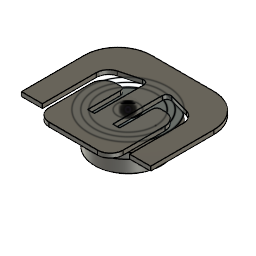
eversweet_pro_3_uvc_base (Autodesk Fusion 360 archive; units mm, degrees)
design "Kitchen Scale Load Cell"
Autodesk Fusion 360 part; units mm, degrees
sketch "Cell" plane through (0, 0, 0) normal (0, 0, 1) x (1, 0, 0)
  line L0 (0, 13) -> (7.4, 13)
  line L1 (15.4, 5) -> (15.4, -10)
  arc A0 (15.4, 5) -> (7.4, 13) centre (7.4, 5) ccw
  line L2 (15.4, -10) -> (10.4, -10)
  line L3 (10.4, -10) -> (10.4, 2.8041)
  line L4 (8.1765, 5.7018) -> (3.4588, 6.9659)
  line L5 (2.2, 6) -> (2.2, -5.8)
  line L6 (2.2, -5.8) -> (3.8, -5.8)
  line L7 (3.8, -5.8) -> (3.8, 2)
  line L8 (4.8, 3) -> (5.8, 3)
  line L9 (8.8, 0) -> (8.8, -10)
  line L10 (5.8, -13) -> (0, -13)
  line L11 (0, -25.6474) -> (0, 25.6474) construction
  arc A1 (10.4, 2.8041) -> (8.1765, 5.7018) centre (7.4, 2.8041) ccw
  arc A2 (5.8, -13) -> (8.8, -10) centre (5.8, -10) ccw
  arc A3 (8.8, 0) -> (5.8, 3) centre (5.8, 0) ccw
  arc A4 (4.8, 3) -> (3.8, 2) centre (4.8, 2) ccw
  arc A5 (3.4588, 6.9659) -> (2.2, 6) centre (3.2, 6) ccw
  line L12 (-5.8, -13) -> (0, -13)
  arc A6 (-8.8, -10) -> (-5.8, -13) centre (-5.8, -10) ccw
  line L13 (-8.8, 0) -> (-8.8, -10)
  arc A7 (-5.8, 3) -> (-8.8, 0) centre (-5.8, 0) ccw
  line L14 (-4.8, 3) -> (-5.8, 3)
  arc A8 (-3.8, 2) -> (-4.8, 3) centre (-4.8, 2) ccw
  line L15 (-3.8, -5.8) -> (-3.8, 2)
  line L16 (-2.2, -5.8) -> (-3.8, -5.8)
  line L17 (-2.2, 6) -> (-2.2, -5.8)
  arc A9 (-2.2, 6) -> (-3.4588, 6.9659) centre (-3.2, 6) ccw
  line L18 (-8.1765, 5.7018) -> (-3.4588, 6.9659)
  arc A10 (-8.1765, 5.7018) -> (-10.4, 2.8041) centre (-7.4, 2.8041) ccw
  line L19 (-10.4, -10) -> (-10.4, 2.8041)
  line L20 (-15.4, -10) -> (-10.4, -10)
  line L21 (-15.4, 5) -> (-15.4, -10)
  arc A11 (-7.4, 13) -> (-15.4, 5) centre (-7.4, 5) ccw
  line L22 (0, 13) -> (-7.4, 13)
  dimension "d3" = 8
  dimension "d4" = 5
  dimension "d7" = 26
  dimension "d8" = 16
  dimension "d9" = 1.6
  dimension "d10" = 1.6
  dimension "d12" = 7.2
  dimension "d13" = 23
  dimension "d14" = 3
  dimension "d15" = 3
  dimension "d16" = 3
  dimension "d17" = 1
  dimension "d18" = 1
  dimension "d19" = 7
  dimension "d20" = 13
  dimension "d21" = 75
  dimension "d22" = 2.2
  dimension "d23" = 5
  constraint horizontal L0
  constraint perpendicular L0 L1
  constraint tangent L0 A0
  constraint tangent L1 A0
  constraint perpendicular L1 L2
  constraint perpendicular L2 L3
  constraint perpendicular L2 L5
  constraint perpendicular L5 L6
  constraint perpendicular L6 L7
  constraint perpendicular L7 L8
  constraint perpendicular L8 L9
  constraint perpendicular L9 L10
  constraint vertical L11
  constraint coincident origin L11
  constraint midpoint origin L11
  constraint coincident L0.start L11
  constraint coincident L10.end L11
  constraint tangent L3 A1
  constraint tangent L4 A1
  constraint tangent L9 A2
  constraint tangent L10 A2
  constraint tangent L8 A3
  constraint tangent L9 A3
  constraint tangent L7 A4
  constraint tangent L8 A4
  constraint tangent L4 A5
  constraint tangent L5 A5
  constraint symmetric L1.end L11 L20.start
  constraint symmetric L0.start L11 L22.start
  constraint symmetric L0.end L11 A11.start
  constraint symmetric L1.start L11 L21.start
  constraint symmetric A0 L11 A11
  constraint symmetric L2.end L11 L19.start
  constraint symmetric L5.end L11 L16.start
  constraint symmetric L6.end L11 L15.start
  constraint symmetric L10.end L11 L12.end
  constraint symmetric L11 L3.end A10.end
  constraint symmetric L11 L4.start L18.start
  constraint symmetric L11 A1 A10
  constraint symmetric L11 L9.end A6.start
  constraint symmetric L11 L10.start L12.start
  constraint symmetric L11 A2 A6
  constraint symmetric L11 L8.end A7.start
  constraint symmetric L11 L9.start L13.start
  constraint symmetric L11 A3 A7
  constraint symmetric L11 L7.end A8.start
  constraint symmetric L11 L8.start L14.start
  constraint symmetric L11 A4 A8
  constraint symmetric L11 L4.end A9.end
  constraint symmetric L11 L5.start L17.start
  constraint symmetric L11 A5 A9
  measures "d3" radius of A0
  measures "d4" distance of L1.end L2.end
  measures "d7" distance of L0 L10
  measures "d8" distance of L8 L10
  measures "d9" distance of L5 L7
  measures "d10" distance of L3 L9
  measures "d12" distance of L6 L10
  measures "d13" distance of L0 L2
  measures "d14" radius of A1
  measures "d15" radius of A2
  measures "d16" radius of A3
  measures "d17" radius of A4
  measures "d18" radius of A5
  measures "d19" distance of L0 A5.centre
  measures "d20" distance of origin L0
  measures "d21" angle of L3 L4
  measures "d22" distance of L5 L11
  measures "d23" distance of L7 L9
extrude "Extrude1" add sketch "Cell" along normal blind 1 makes body 1
sketch "Foot" plane through (0, 0, 0) normal (0, 0, 1) x (1, 0, 0)
  circle A0 centre (0, 0) radius 7.95
  circle A1 centre (0, 0) radius 9.45
  circle A2 centre (0, 0) radius 6.6
  circle A3 centre (0, 0) radius 2.5
  dimension "d26" = 15.9
  dimension "d27" = 18.9
  dimension "d28" = 13.2
  dimension "d29" = 5
  constraint coincident A0.centre A1.centre
  constraint concentric A0 A1
  constraint concentric A0 A2
  constraint concentric A2 A3
  measures "d26" diameter of A0
  measures "d27" diameter of A1
  measures "d28" diameter of A2
  measures "d29" diameter of A3
extrude "Extrude2" add sketch "Foot" against normal blind 3.6 separate body contours A3 makes body 2
extrude "Extrude3" add sketch "Foot" along normal blind 1.4 from surface at -3.6 contours A0 | A1 | A2 bodies 2
extrude "Extrude4" add sketch "Foot" against normal blind 4 from surface at -3.6 contours A0 | A2 | A3 bodies 2
extrude "Extrude5" add sketch "Foot" against normal blind 1 from surface at -7.6 contours A2 | A3 bodies 2
equation "d22 = ( 4.4 / 2 ) * 1 mm"
named bodies: "Cell", "Foot"
